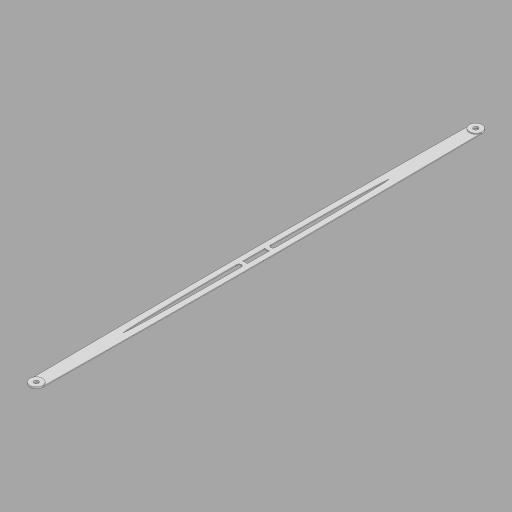
# Autodesk Inventor part: szalag3
Saved by Autodesk Inventor 2023 (Build 270158000, 158)
## iProperties
Created: 2022-11-15
Part Number: szalag3
Material: Generic
Document SubType Name: Modeling
Designer: gd1
Density: 1 g/cm^3
Appearance: Default
Mass: 8.05587 g
Surface Area: 174.106 cm^2
Volume: 8.05587 cm^3
Author: gd1
Autodesk Inventor part; units mm, degrees
ref_plane "YZ Plane" through (0, 0, 0) normal (1, 0, 0) x (0, 1, 0)
ref_plane "XZ Plane" through (0, 0, 0) normal (0, 1, 0) x (-1, 0, 0)
ref_plane "XY Plane" through (0, 0, 0) normal (0, 0, 1) x (1, 0, 0)
sketch "Sketch1" plane through (0, 0, 0) normal (0, 1, 0) x (-1, 0, 0)
  line L0 (0, 0) -> (0, -244.423)
  line L1 (0, 0) -> (244.423, 0) construction
  line L2 (0, -244.423) -> (0, -285.4289)
  line L3 (0, -285.4289) -> (0, -529.8519)
  circle A0 centre (0, -244.423) radius 2.75
  circle A1 centre (0, -285.4289) radius 2.75
  circle A2 centre (0, 0) radius 2.75
  circle A3 centre (0, 0) radius 7.5
  circle A4 centre (0, -529.8519) radius 7.5
  circle A5 centre (0, -264.9259) radius 9
  spline S0 degree 2 poles (7.5, 0) (10.5, -264.9259) (7.5, -529.8519) knots 0 0 0 1 1 1
  spline S1 degree 2 poles (-7.5, -529.8519) (-10.5, -264.9259) (-7.5, 0) knots 0 0 0 1 1 1
  ellipse E0 centre (0, -264.9259) end of major axis (0, -104.9259) minor radius 2.7588
  circle A6 centre (0, -529.8519) radius 2.75
  circle A7 centre (0, -244.423) radius 7.5
  circle A8 centre (0, -285.4289) radius 7.5
  line L4 (7.5, -285.4289) -> (-7.5, -285.4289)
  line L5 (7.5, -244.423) -> (-7.5, -244.423)
  point P0 (9, -264.9259)
  point P1 (-9, -264.9259)
  point P2 (0, -522.3519)
  point P3 (0, -7.5)
  point P4 (-2.7354, -244.1399)
  point P5 (2.7354, -244.1399)
  point P6 (2.7366, -244.694)
  point P7 (2.7548, -256.3579)
  point P8 (-2.7548, -256.3579)
  point P9 (-2.7366, -244.694)
  point P10 (2.7548, -273.494)
  point P11 (2.7366, -285.1579)
  point P12 (2.7354, -285.712)
  point P13 (-2.7354, -285.712)
  point P14 (-2.7366, -285.1579)
  point P15 (-2.7548, -273.494)
  point P16 (2.7489, -278.4508)
  point P17 (-2.7489, -278.4508)
  point P18 (2.7489, -251.4011)
  point P19 (-2.7489, -251.4011)
  dimension "d15" = 160
  dimension "d0" = 244.423
  dimension "d1" = 90
  dimension "d2" = 41.0059
  dimension "d3" = 244.423
  dimension "d4" = 5.5
  dimension "d5" = 5.5
  dimension "d6" = 5.5
  dimension "d7" = 15
  dimension "d8" = 15
  dimension "d9" = 18
  dimension "d10" = 5.5
  dimension "d16" = 15
  dimension "d17" = 15
  constraints: 12 end point, 10 point on circle, 9 centre point, 9 coincident, 3 vertical, 2 horizontal, 1 midpoint, 1 parallel, 1 perpendicular, 1 point on line, 8 other
  measures "d0" distance of L0.start L0.end
  measures "d1" angle of L0 L1
  measures "d2" distance of L0.end L2.end
  measures "d3" distance of L2.end L3.end
  measures "d4" diameter of A0
  measures "d5" diameter of A1
  measures "d6" diameter of A2
  measures "d7" diameter of A3
  measures "d8" diameter of A4
  measures "d9" diameter of A5
  measures "d10" diameter of A6
  measures "d16" diameter of A7
  measures "d17" diameter of A8
extrude "Extrusion1" add sketch "Sketch1" along normal blind 2 contours A3 | A4
extrude "Extrusion2" add sketch "Sketch1" along normal blind 1 contours A3 S0 A5 E0 A7 L0 | L0 E0 A7 A5 S1 A3 | E0 A0 L5 A7 | A7 L5 A0 E0 | A5 E0 | A5 E0 A8 L3 A4 S1 | A5 E0 | S0 A4 L3 E0 A8 A5 | L5 A0 E0 A7 | A7 E0 A0 L5 | E0 A1 L4 A8 | A8 L4 A1 E0 | L4 A1 E0 A8 | A8 E0 A1 L4
extrude "Extrusion3" add sketch "Sketch1" along normal blind 1 contours E0 A0 L2 A7 | A7 L2 A0 E0 | A8 L2 A1 E0 | E0 A1 L2 A8
body "Solid1"
